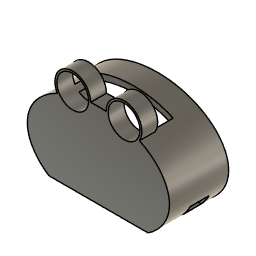
CASA0014-v1.0 (Autodesk Fusion 360 design; units mm, degrees)
Autodesk Fusion 360 part; units mm, degrees
sketch "Sketch1" plane through (0, 0, 0) normal (0, 1, 0) x (1, 0, 0)
  circle A0 centre (13, 0) radius 8.05
  circle A1 centre (-13, 0) radius 8.05
  circle A2 centre (13, 0) radius 9.05
  circle A3 centre (-13, 0) radius 9.05
  ellipse E0 centre (0, 25) end of major axis (0, 0) minor radius 36
  line L0 (0, 50) -> (0, 0) construction
  line L1 (-36, 25) -> (36, 25) construction
  line L2 (-25.1369, 42.8964) -> (25.1369, 42.8964)
  spline S0 degree 3 poles (-33, 25) (-33, 21.436) (-31.6665, 17.8323) (-28.9735, 14.5432) (-26.2575, 11.2263) (-22.141, 8.2837) (-17.1368, 6.2364) (-11.7492, 4.0324) (-5.3608, 2.8822) (0.9825, 3.0099) (7.2458, 3.1359) (13.4399, 4.5067) (18.5764, 6.8602) (23.2376, 8.9959) (27.0077, 11.9255) (29.4645, 15.1662) (32.1222, 18.672) (33.2689, 22.482) (32.9473, 26.2304) (32.646, 29.7421) (31.0347, 33.2754) (28.117, 36.4419) (25.1302, 39.6833) (20.7686, 42.4875) (15.5971, 44.3561) (9.9796, 46.3859) (3.434, 47.2975) (-2.9473, 46.9109) (-9.0671, 46.5401) (-15.0119, 44.9789) (-19.8696, 42.5163) (-24.5363, 40.1505) (-28.1733, 36.9711) (-30.3729, 33.5325) (-32.1337, 30.7797) (-33, 27.8816) (-33, 25) knots -3.141593 -3.141593 -3.141593 -3.141593 -2.62457 -2.62457 -2.62457 -2.103164 -2.103164 -2.103164 -1.541824 -1.541824 -1.541824 -0.987565 -0.987565 -0.987565 -0.484591 -0.484591 -0.484591 0.059511 0.059511 0.059511 0.569241 0.569241 0.569241 1.091031 1.091031 1.091031 1.657814 1.657814 1.657814 2.201379 2.201379 2.201379 2.723562 2.723562 2.723562 3.141593 3.141593 3.141593 3.141593
  line L3 (-25.1369, 39.8964) -> (25.1369, 39.8964)
  dimension "d1" = 13
  dimension "d2" = 13
  dimension "d3" = 16.1
  dimension "d4" = 16.1
  dimension "d5" = 1
  dimension "d6" = 1
  dimension "d7" = 72
  dimension "d8" = -3
  dimension "d9" = 3
  constraint coincident E0 L0.start
  constraint coincident E0 L0.end
  constraint coincident E0 L1.start
  constraint coincident E0 L1.end
  constraint coincident L0.end origin
  constraint vertical L0
  constraint coincident E0 L2.start
  constraint coincident E0 L2.end
  constraint perpendicular L0 L2
  measures "d1" distance of L0.end A0.centre
  measures "d2" distance of L0.end A1.centre
  measures "d3" diameter of A0
  measures "d4" diameter of A1
extrude "Extrude1" add sketch "Sketch1" along normal blind 30 contours A2 E0 L2 S0 | L2 S0 L3 | A3 E0 L2 S0 makes body 1
extrude "Extrude2" add sketch "Sketch1" along normal blind 8 contours A1 A3 S0 bodies 1
extrude "Extrude3" add sketch "Sketch1" along normal blind 8 separate body contours A0 A2 E0 makes body 2
extrude "Extrude4" add sketch "Sketch1" along normal blind 8 contours A0 A2 E0 S0 | A0 A2 E0 S0 | A0 A2 S0 bodies 1 2
extrude "Extrude5" add sketch "Sketch1" along normal blind 8 separate body contours A2 A3 E0 S0 makes body 3
extrude "Extrude6" add sketch "Sketch1" along normal blind 8 contours A1 A3 E0 S0 | A1 A3 E0 | A1 A3 E0 S0 bodies 1 3
extrude "Extrude7" cut sketch "Sketch1" along normal blind 30 contours A0 E0 S0 | A0 A2 E0 S0 | A0 A2 E0 S0 | A2 A3 E0 S0 | A1 A3 E0 S0 | A1 E0 S0 | A1 A3 E0 S0 bodies 1
extrude "Extrude8" add sketch "Sketch1" along normal blind 30 contours A0 E0 S0 | A0 A2 E0 S0 | A0 A2 E0 S0 | A2 A3 E0 S0 | A1 A3 E0 S0 | A1 E0 S0 | A1 A3 E0 S0 bodies 1
extrude "Extrude9" add sketch "Sketch1" along normal blind 4 contours A2 A3 S0 L3 bodies 1
extrude "Extrude10" cut sketch "Sketch1" along normal blind 18 contours A1 E0 S0 bodies 1
extrude "Extrude11" cut sketch "Sketch1" along normal blind 18 contours A0 E0 S0 bodies 1
sketch "Sketch2" plane through (0, 0, 0) normal (0, 0, 1) x (1, 0, 0)
  line L0 (-12, 18) -> (12, 18)
  line L1 (12, 18) -> (12, 8)
  line L2 (12, 8) -> (-12, 8)
  line L3 (-12, 8) -> (-12, 18)
  constraint horizontal L0
  constraint vertical L1
  constraint horizontal L2
  constraint vertical L3
extrude "Extrude12" cut sketch "Sketch2" against normal blind 10 bodies 1
sketch "Sketch3" plane through (0, 0, 0) normal (1, 0, 0) x (0, 1, 0)
  line L0 (12.5, -38.6504) -> (22, -38.6504)
  line L1 (22, -38.6504) -> (22, -33.1504)
  line L2 (22, -33.1504) -> (12.5, -33.1504)
  line L3 (12.5, -33.1504) -> (12.5, -38.6504)
  dimension "d36" = 5.5
  constraint horizontal L0
  constraint vertical L1
  constraint horizontal L2
  constraint vertical L3
  measures "d36" distance of L0.start L2.end
extrude "Extrude13" cut sketch "Sketch3" along normal blind 40 bodies 1
sketch "Sketch4" plane through (0, 30, 0) normal (0, 1, 0) x (-1, 0, 0)
  ellipse E0 centre (0, -25) end of major axis (-36, -25) minor radius 25 (25.1369, -42.8964) -> (-25.1369, -42.8964) ccw
  line L0 (-25.1369, -42.8964) -> (25.1369, -42.8964)
  spline S0 degree 3 poles (-18.7874, -6.9576) (-18.7173, -6.925) (-18.6469, -6.8925) (-18.5764, -6.8602) (-18.3054, -6.736) (-18.0314, -6.6145) (-17.7546, -6.4958) knots 0.979955 0.979955 0.979955 0.979955 0.987565 0.987565 0.987565 1.016811 1.016811 1.016811 1.016811
  spline S1 degree 3 poles (-17.7546, -6.4958) (-14.1037, -4.9304) (-9.9657, -3.8479) (-5.6739, -3.3364) knots 1.016811 1.016811 1.016811 1.016811 1.402589 1.402589 1.402589 1.402589
  spline S2 degree 3 poles (-5.6739, -3.3364) (-5.2972, -3.2915) (-4.9192, -3.251) (-4.5403, -3.2149) knots 1.402589 1.402589 1.402589 1.402589 1.436456 1.436456 1.436456 1.436456
  spline S3 degree 3 poles (-4.5403, -3.2149) (-3.3614, -3.1028) (-2.1732, -3.0338) (-0.9825, -3.0099) (0.8635, -2.9727) (2.7134, -3.0438) (4.5413, -3.2176) knots 1.436456 1.436456 1.436456 1.436456 1.541824 1.541824 1.541824 1.705185 1.705185 1.705185 1.705185
  spline S4 degree 3 poles (4.5413, -3.2176) (4.9202, -3.2536) (5.2982, -3.294) (5.6751, -3.3389) knots 1.705185 1.705185 1.705185 1.705185 1.739052 1.739052 1.739052 1.739052
  spline S5 degree 3 poles (5.6751, -3.3389) (9.7264, -3.8206) (13.6422, -4.8068) (17.1368, -6.2364) (17.3443, -6.3213) (17.5503, -6.4078) (17.7548, -6.4957) knots 1.739052 1.739052 1.739052 1.739052 2.103164 2.103164 2.103164 2.124788 2.124788 2.124788 2.124788
  spline S6 degree 3 poles (17.7548, -6.4957) (18.1033, -6.6457) (18.4472, -6.7999) (18.7865, -6.9584) knots 2.124788 2.124788 2.124788 2.124788 2.161648 2.161648 2.161648 2.161648
  spline S7 degree 3 poles (18.7865, -6.9584) (23.0469, -8.9485) (26.5622, -11.5984) (28.9735, -14.5432) (31.6665, -17.8323) (33, -21.436) (33, -25) (33, -27.8816) (32.1337, -30.7797) (30.3729, -33.5325) (28.9074, -35.8235) (26.8038, -37.9995) (24.1827, -39.8964) knots -4.121537 -4.121537 -4.121537 -4.121537 -3.658615 -3.658615 -3.658615 -3.141593 -3.141593 -3.141593 -2.723562 -2.723562 -2.723562 -2.37565 -2.37565 -2.37565 -2.37565
  line L1 (24.1827, -39.8964) -> (-24.1808, -39.8964)
  spline S8 degree 3 poles (-24.1808, -39.8964) (-25.6682, -38.8249) (-26.9904, -37.6645) (-28.117, -36.4419) (-31.0347, -33.2754) (-32.646, -29.7421) (-32.9473, -26.2304) (-33.2689, -22.482) (-32.1222, -18.672) (-29.4645, -15.1662) (-27.0448, -11.9745) (-23.3514, -9.0846) (-18.7874, -6.9576) knots -0.766054 -0.766054 -0.766054 -0.766054 -0.569241 -0.569241 -0.569241 -0.059511 -0.059511 -0.059511 0.484591 0.484591 0.484591 0.979955 0.979955 0.979955 0.979955
  line L2 (-26.6711, -12.125) -> (26.6722, -12.125)
  constraint coincident S8 L2.start
  constraint coincident S7 L2.end
  constraint horizontal L2
copy_body "CopyPasteBodies1" bodies 1 makes body 4
move_body "Move1" bodies 4 to x (1, 0, 0) y (0, 0, 1) z (0, -1, 0) at (0, -42.8964, -42.8964)
hidden bodies 4
